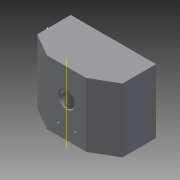
# Autodesk Inventor part: odorport_final_wvac
Saved by Autodesk Inventor 2015 SP1 (Build 190203100, 203)
## iProperties
Created: 2014-11-21
Part Number: odorport_final_wvac
Material: Generic
Document SubType Name: Modeling
Designer: cdw291
Density: 1 g/cm^3
Appearance: Default
Author: cdw291
Autodesk Inventor part; units mm, degrees
ref_plane "YZ Plane" through (0, 0, 0) normal (1, 0, 0) x (0, 1, 0)
ref_plane "XZ Plane" through (0, 0, 0) normal (0, 1, 0) x (-1, 0, 0)
ref_plane "XY Plane" through (0, 0, 0) normal (0, 0, 1) x (1, 0, 0)
sketch "Sketch1" plane through (0, 0, 0) normal (0, 1, 0) x (-1, 0, 0)
  line L0 (12.7, 6.985) -> (-12.7, 6.985)
  line L1 (-12.7, 6.985) -> (-12.7, -6.985)
  line L2 (-12.7, -6.985) -> (12.7, -6.985)
  line L3 (12.7, -6.985) -> (12.7, 6.985)
  point P0 (0, 0)
  dimension "depth" = 25.4
  dimension "width" = 13.97
  dimension "d5" = 6.985
  dimension "d6" = 12.7
  constraints: 8 end point, 2 parallel, 1 horizontal, 1 perpendicular
  measures "depth" distance between parallel lines of L1 L3
  measures "width" distance between parallel lines of L2 L0
  measures "d5" distance from line of L0 point (0, 0)
  measures "d6" distance from line of L1 point (0, 0)
extrude "body" add sketch "Sketch1" along normal blind 19.05
sketch "Sketch3" plane through (12.7, 0, 6.985) normal (1, 0, 0) x (0, 0, -1)
  point P0 (6.985, 0)
sketch "Sketch5" plane through (0, 19.05, 0) normal (0, 1, 0) x (1, 0, 0)
  line L0 (-12.7, -6.985) -> (12.7, -6.985) projected
  point P0 (0, 0)
  point P1 (0, -4.699)
  dimension "d25" = 0
  dimension "d34" = 6.985
  dimension "hole_radius" = 2.286
  measures "d25" horizontal distance of point (0, 0) point (0, -4.699)
  measures "d34" distance from line of L0 point (0, 0)
  measures "hole_radius" distance from line of L0 point (0, -4.699)
hole "main odor hole" at (0, 19.05, 4.699) direction (0, -1, 0) diameter 4.2291 depth 14.732 tip angle 118
sketch "Sketch6" plane through (-12.7, 0, 6.985) normal (0, 0, 1) x (1, 0, 0)
  line L0 (0, 0) -> (25.4, 0) projected
  point P0 (12.7, 0)
  point P1 (15.2082, 15.494)
  point P2 (10.1917, 15.494)
  dimension "d126" = 15.494
  dimension "d127" = 5.0165
  dimension "d128" = 2.5082
  constraints: 1 horizontal alignment
  measures "d126" distance from line of L0 point (15.208, 15.494)
  measures "d127" distance of point (10.192, 15.494) point (15.208, 15.494)
  measures "d128" horizontal distance of point (12.7, 0) point (10.192, 15.494)
hole "lickports" at (2.5083, 15.494, 6.985) at (-2.5082, 15.494, 6.985) direction (0, 0, -1) diameter 0.7112 end through all
sketch "Sketch7" plane through (12.7, 0, -6.985) normal (0, 0, -1) x (-1, 0, 0)
  line L0 (14.8146, 4.318) -> (10.5855, 4.318) projected
  point P0 (12.7, 0)
  point P1 (12.7, 4.318)
  constraints: 1 midpoint
hole "fitting threads" at (0, 4.318, -6.985) direction (0, 0, 1) diameter 5.3594 depth 6.35 thread size "1/4-28 UNF" class "2B" standard "ANSI Unified Screw Threads"
sketch "Sketch8" plane through (0, 4.318, -0.635) normal (0, 0, -1) x (-1, 0, 0)
  line L0 (2.1146, 0) -> (-2.1145, 0) projected
  point P0 (0, -4.318)
  point P1 (0, 0)
  constraints: 1 midpoint
hole "input odor hole" at (0, 4.318, -0.635) direction (0, 0, 1) diameter 0.7937 depth 5.08
sketch "Sketch9" plane through (-12.7, 0, 6.985) normal (0, 0, 1) x (1, 0, 0)
  line L0 (0, 0) -> (25.4, 0) projected
  point P0 (12.7, 0)
  point P1 (12.7, 8.636)
  point P2 (12.7, 0)
  dimension "nose_hole" = 8.636
  constraints: 1 midpoint, 1 vertical alignment
  measures "nose_hole" distance from line of L0 point (12.7, 8.636)
hole "nose_hole" at (0, 8.636, 6.985) direction (0, 0, -1) diameter 4.445 depth 4.1148 tip angle 110
sketch "Sketch10" plane through (0, 19.05, 0) normal (0, 1, 0) x (1, 0, 0)
  point P0 (0, 0)
  point P1 (7.9375, 2.54)
  point P2 (-7.9375, 2.54)
  dimension "d70" = 2.54
  dimension "d116" = 15.875
  dimension "d117" = 7.9375
  constraints: 1 horizontal alignment
  measures "d70" vertical distance of point (7.937, 2.54) point (0, 0)
  measures "d116" distance of point (7.937, 2.54) point (-7.938, 2.54)
  measures "d117" horizontal distance of point (7.937, 2.54) point (0, 0)
hole "mount holes" at (7.9375, 19.05, -2.54) at (-7.9375, 19.05, -2.54) direction (0, -1, 0) diameter 2.6416 depth 10.16 tip angle 118 thread size "6-32 UNC" class "2B" standard "ANSI Unified Screw Threads"
sketch "Sketch11" plane through (12.7, 0, -6.985) normal (0, 0, -1) x (-1, 0, 0)
  line L0 (0, 19.05) -> (25.4, 19.05) projected
  line L1 (0, 0) -> (25.4, 0) projected
  point P0 (12.7, 0)
  point P1 (12.7, 13.208)
  point P2 (12.7, 0)
  dimension "vacuum_height" = 5.842
  constraints: 1 midpoint, 1 vertical alignment
  measures "vacuum_height" distance from line of L0 point (12.7, 13.208)
hole "exhaust threading" at (0, 13.208, -6.985) direction (0, 0, 1) diameter 3.9624 depth 6.35 thread size "10-32 UNF" class "2B" standard "ANSI Unified Screw Threads"
sketch "Sketch12" plane through (0, 13.208, -0.635) normal (0, 0, -1) x (-1, 0, 0)
  line L0 (-12.7, -13.208) -> (12.7, -13.208) projected
  line L1 (-12.7, 5.842) -> (12.7, 5.842) projected
  point P0 (0, -13.208)
  point P1 (0, 0)
  point P2 (0, -13.208)
  dimension "d87" = 5.842
  constraints: 1 midpoint, 1 vertical alignment
  measures "d87" distance from line of L1 point (0, 0)
hole "exhaust hole" at (0, 13.208, -0.635) direction (0, 0, 1) diameter 1.5875 depth 5.08
sketch "Sketch16" plane through (12.7, 0, -6.985) normal (0, 0, -1) x (-1, 0, 0)
  circle A0 centre (12.7, 8.636) radius 2.9083 projected
  line L0 (15.6083, 8.636) -> (12.7, 8.636)
  point P0 (12.7, 0)
  constraints: 2 end point, 1 coincident, 1 horizontal, 1 horizontal alignment, 1 other
hole "sniff_monitoring_hole" at (0, 8.636, -6.985) direction (0, 0, 1) diameter 0.7112 end through all
fillet "nose hole fillet" [suppressed]
sketch "Sketch25" plane through (12.7, 0, 6.985) normal (1, 0, 0) x (0, 0, -1)
  line L0 (7.62, 1.6383) -> (7.62, 6.9977) projected
  point P0 (6.985, 0)
  point P1 (7.62, 4.318)
  point P2 (6.5343, 4.318)
  point P3 (4.363, 4.318)
  dimension "d147" = 3.257
  dimension "d148" = 1.0857
  constraints: 1 horizontal alignment, 1 midpoint
  measures "d147" distance of point (4.363, 4.318) point (7.62, 4.318)
  measures "d148" distance of point (7.62, 4.318) point (6.534, 4.318)
hole "vac fitting" at (12.7, 4.318, 0.4507) direction (-1, 0, 0) diameter 3.9624 depth 6.35 thread size "10-32 UNF" class "2B" standard "ANSI Unified Screw Threads"
hole "vac hole" at (6.35, 4.318, 0.4507) direction (-1, 0, 0) diameter 0.7937 depth 6.35 tip angle 118
chamfer "front panel chamfer" distance 6.858 angle 30 2 edges at (12.7, 9.525, 6.985) (-12.7, 9.525, 6.985) measured on face at (9.2021, 9.318, 6.985)
fillet "Fillet4" radius 0.381 1 edges at (0, 10.8585, 6.985)
equation "\"d5\" = 0.5 * width"
equation "\"d6\" = 0.5 * depth"
equation "\"d27\" = 1.85 * hole_radius"
equation "\"d29\" = 2 * hole_radius"
equation "\"d127\" = 2 * hole_radius + 0.625 * lick_port_diam"
equation "\"d128\" = 0.5 * d127"
equation "\"d66\" = 1.8 * hole_radius"
equation "\"d117\" = 0.5 * d116"
equation "\"d87\" = vacuum_height"
equation "\"d148\" = 0.333333 * d147"
equation "\"d150\" = vac_thread_depth"
equation "\"d154\" = vac_fit_depth"
equation "\"vac_thread_depth\" = 5.08"
equation "\"vac_fit_depth\" = 6.35"
equation "\"lick_port_diam\" = 0.7112"
body "Solid1"
